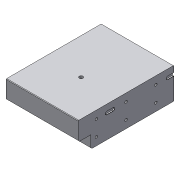
# Autodesk Inventor part: BC-10010
Saved by Autodesk Inventor 2016 (Build 200138000, 138)
## iProperties
Created: 2015-10-07
Part Number: BC-10010
Project: DIPOLO BC-3T- SIRIUS
Cost Center: 1504002005
Material: Alumínio 7075
Document SubType Name: Modeling
Designer: reinaldo.basilio
Mass: 37073.4 g
Surface Area: 4103.36 cm^2
Volume: 13193.4 cm^3
Density: 2.81 g/cm^3
Appearance: Aluminum - Flat
Description: Espaçador da metade superior e inferior do dipolo.
RuleStatus: InUse
AfterMaterialChange0: file://_iMaterial
AfterAnyiPropertyChange0: file://_iMaterial
AfterDocNew0: file://_Naming_par
AfterDocNew1: file://_NameStart
AfterDocNew2: file://_NameStart1
AfterDocNew3: file://_Materiais
DocNumber: XXXXX-XXX-XXXX-00-001.ipt
Folder: .
Title: DIPOLO BC-3T- SIRIUS
Author: reinaldo.basilio
Subject: BC-10010
Autodesk Inventor part; units mm, degrees
ref_plane "YZ Plane" through (0, 0, 0) normal (1, 0, 0) x (0, 1, 0)
ref_plane "XZ Plane" through (0, 0, 0) normal (0, 1, 0) x (-1, 0, 0)
ref_plane "XY Plane" through (0, 0, 0) normal (0, 0, 1) x (1, 0, 0)
sketch "Sketch5" plane through (0, 0, 0) normal (0, 1, 0) x (-1, 0, 0)
  line L0 (452.5, 48) -> (452.5, 173)
  line L1 (117.5, 98) -> (117.5, 48)
  line L2 (117.5, 48) -> (452.5, 48)
  line L3 (67.5, 173) -> (67.5, 98)
  line L4 (67.5, 98) -> (117.5, 98)
  line L5 (67.5, 173) -> (452.5, 173)
  dimension "d8" = 125
  dimension "d13" = 385
  dimension "d18" = 50
  dimension "d42" = 50
  constraints: 12 end point, 2 horizontal, 2 perpendicular, 2 vertical
  measures "d8" distance of L0.start L0.end
  measures "d13" distance of L3.start L0.end
  measures "d18" distance of L1.start L1.end
  measures "d42" distance of L3.end L1.start
extrude "Extrusion5" add sketch "Sketch5" along normal blind 291
sketch "Sketch6" plane through (0, 291, 0) normal (0, 1, 0) x (1, 0, 0)
  line L0 (-452.5, -173) -> (-67.5, -173) projected
  line L1 (-117.5, -48) -> (-452.5, -48) projected
  circle A0 centre (-140, -141.75) radius 6
  circle A1 centre (-140, -79.25) radius 6
  circle A2 centre (-260, -141.75) radius 6
  circle A3 centre (-260, -79.25) radius 6
  circle A4 centre (-380, -141.75) radius 6
  circle A5 centre (-380, -79.25) radius 6
  line L2 (-452.5, -48) -> (-452.5, -173) projected
  line L3 (-67.5, -173) -> (-67.5, -98) projected
  point P0 (0, 0)
  point P1 (-260, -173)
  dimension "d19" = 12
  dimension "d20" = 120
  dimension "d21" = 385
  dimension "d22" = 125
  dimension "d23" = 120
  dimension "d24" = 62.5
  dimension "d25" = 31.25
  dimension "d26" = 31.25
  dimension "d41" = 72.5
  dimension "d61" = 72.5
  dimension "d62" = 192.5
  constraints: 6 centre point, 5 equal radius, 4 horizontal alignment, 4 vertical alignment, 1 midpoint
  measures "d19" diameter of A0
  measures "d20" distance of A2.centre A0.centre
  measures "d21" distance of L0.start L0.end
  measures "d22" distance of L1.end L0.start
  measures "d23" distance of A4.centre A2.centre
  measures "d24" distance of A5.centre A4.centre
  measures "d25" distance from line of L0 A4.centre
  measures "d26" distance from line of L1 A5.centre
  measures "d41" distance from line of L2 A4.centre
  measures "d61" distance from line of L3 A0.centre
  measures "d62" distance from line of A3.centre L2
hole "Hole1" at (-140, 291, 141.75) at (-260, 291, 141.75) at (-380, 291, 141.75) at (-380, 291, 79.25) at (-260, 291, 79.25) at (-140, 291, 79.25) direction (0, -1, 0) diameter 10.106 depth 35 tip angle 118 thread size "M12x1.75" class "6H" standard "ISO Metric profile"
sketch "Sketch7" plane through (0, 0, 0) normal (0, -1, 0) x (1, 0, 0)
  circle A0 centre (-380, 141.75) radius 5.053
  circle A1 centre (-380, 79.25) radius 5.053
  circle A2 centre (-260, 141.75) radius 5.053
  circle A3 centre (-260, 79.25) radius 5.053
  circle A4 centre (-140, 141.75) radius 5.053
  circle A5 centre (-140, 79.25) radius 5.053
  circle A6 centre (-140, 141.75) radius 5.053 projected
  circle A7 centre (-140, 79.25) radius 5.053 projected
  circle A8 centre (-260, 79.25) radius 5.053 projected
  circle A9 centre (-260, 141.75) radius 5.053 projected
  circle A10 centre (-380, 141.75) radius 5.053 projected
  circle A11 centre (-380, 79.25) radius 5.053 projected
  point P0 (0, 0)
  constraints: 12 concentric, 6 centre point
hole "Hole2" at (-380, 0, 141.75) at (-380, 0, 79.25) at (-260, 0, 79.25) at (-260, 0, 141.75) at (-140, 0, 141.75) at (-140, 0, 79.25) direction (0, 1, 0) diameter 10.106 depth 35 tip angle 118 thread size "M12x1.75" class "6H" standard "ISO Metric profile"
chamfer "Chamfer1" distance 5 angle 45 2 edges at (-67.5, 145.5, 98) (-117.5, 145.5, 48)
sketch "Sketch8" plane through (0, 291, 0) normal (0, 1, 0) x (1, 0, 0)
  line L0 (-182.5, -141.75) -> (-207.5, -141.75) construction
  line L1 (-182.5, -135.75) -> (-207.5, -135.75)
  line L2 (-207.5, -147.75) -> (-182.5, -147.75)
  arc A0 (-182.5, -147.75) -> (-182.5, -135.75) centre (-182.5, -141.75) ccw
  arc A1 (-207.5, -135.75) -> (-207.5, -147.75) centre (-207.5, -141.75) ccw
  line L3 (-427.5, -141.75) -> (-452.5, -141.75) construction
  line L4 (-427.5, -135.75) -> (-452.5, -135.75)
  line L5 (-452.5, -147.75) -> (-427.5, -147.75)
  arc A2 (-427.5, -147.75) -> (-427.5, -135.75) centre (-427.5, -141.75) ccw
  arc A3 (-452.5, -135.75) -> (-452.5, -147.75) centre (-452.5, -141.75) ccw
  line L6 (-452.5, -48) -> (-452.5, -173) projected
  circle A4 centre (-260, -141.75) radius 5.053 projected
  point P0 (0, 0)
  point P1 (-440, -141.75)
  point P2 (-195, -141.75)
  point P3 (-440, -141.75)
  point P4 (-195, -147.75)
  point P5 (-195, -141.75)
  dimension "d46" = 12
  dimension "d47" = 12
  dimension "d48" = 25
  dimension "d49" = 25
  dimension "d58" = 12.5
  dimension "d60" = 257.5
  constraints: 16 end point, 8 point on circle, 8 tangent, 4 centre point, 4 midpoint, 2 parallel, 2 point on line, 1 coincident, 1 horizontal, 1 horizontal alignment, 1 vertical alignment
  measures "d46" distance between parallel lines of L1 L2
  measures "d47" distance between parallel lines of L4 L5
  measures "d48" distance of L0.start L0.end
  measures "d49" distance of L3.start L3.end
  measures "d58" distance from line of L6 point (-440, -141.75)
  measures "d60" distance from line of L6 point (-195, -141.75)
extrude "Extrusion6" cut sketch "Sketch8" against normal blind 5 contours A0 L2 A1 L1 | A2 L5 L6 L4 | L6 A3
sketch "Sketch9" plane through (0, 0, 0) normal (0, -1, 0) x (1, 0, 0)
  line L0 (-452.5, 141.75) -> (-427.5, 141.75) construction
  line L1 (-452.5, 135.75) -> (-427.5, 135.75)
  line L2 (-427.5, 147.75) -> (-452.5, 147.75)
  arc A0 (-452.5, 147.75) -> (-452.5, 135.75) centre (-452.5, 141.75) ccw
  arc A1 (-427.5, 135.75) -> (-427.5, 147.75) centre (-427.5, 141.75) ccw
  line L3 (-207.5, 141.75) -> (-182.5, 141.75) construction
  line L4 (-207.5, 135.75) -> (-182.5, 135.75)
  line L5 (-182.5, 147.75) -> (-207.5, 147.75)
  arc A2 (-207.5, 147.75) -> (-207.5, 135.75) centre (-207.5, 141.75) ccw
  arc A3 (-182.5, 135.75) -> (-182.5, 147.75) centre (-182.5, 141.75) ccw
  arc A4 (-427.5, 135.75) -> (-427.5, 147.75) centre (-427.5, 141.75) ccw projected
  arc A5 (-207.5, 147.75) -> (-207.5, 135.75) centre (-207.5, 141.75) ccw projected
  arc A6 (-182.5, 135.75) -> (-182.5, 147.75) centre (-182.5, 141.75) ccw projected
  line L6 (-452.5, 48) -> (-452.5, 173) projected
  point P0 (0, 0)
  point P1 (-440, 141.75)
  point P2 (-195, 141.75)
  dimension "d76" = 25
  dimension "d77" = 25
  dimension "d78" = 12.5
  constraints: 16 end point, 8 point on circle, 8 tangent, 4 centre point, 4 concentric, 2 midpoint, 2 parallel, 2 point on line, 1 horizontal
  measures "d76" distance of L3.start L3.end
  measures "d77" distance of L0.start L0.end
  measures "d78" distance from line of point (-440, 141.75) L6
extrude "Extrusion7" cut sketch "Sketch9" against normal blind 5
sketch "Sketch10" plane through (-452.5, 0, 48) normal (0, 0, -1) x (-1, 0, 0)
  line L0 (0, 0) -> (0, 291) projected
  line L1 (-330, 291) -> (0, 291) projected
  circle A0 centre (-295, 145.5) radius 5
  circle A1 centre (-165, 145.5) radius 5
  circle A2 centre (-35, 145.5) radius 5
  point P0 (-452.5, 0)
  point P1 (0, 145.5)
  point P2 (-165, 291)
  dimension "d63" = 130
  dimension "d64" = 130
  dimension "d65" = 10
  constraints: 3 centre point, 3 horizontal alignment, 2 equal radius, 2 midpoint, 1 vertical alignment
  measures "d63" distance of A1.centre A0.centre
  measures "d64" distance of A2.centre A1.centre
  measures "d65" diameter of A0
hole "Hole3" at (-157.5, 145.5, 48) at (-287.5, 145.5, 48) at (-417.5, 145.5, 48) direction (0, 0, 1) diameter 8.376 depth 25 tip angle 118 thread size "M10x1.5" class "6H" standard "ISO Metric profile"
chamfer "Chamfer2" distance 0.5 angle 45 14 edges at (-195, 291, 147.75) (-213.5, 291, 141.75) (-195, 291, 135.75) (-176.5, 291, 141.75) (-440, 291, 147.75) (-440, 291, 135.75) (-421.5, 291, 141.75) (-213.5, 0, 141.75) (-195, 0, 147.75) (-176.5, 0, 141.75) (-195, 0, 135.75) (-440, 0, 147.75) (-421.5, 0, 141.75) (-440, 0, 135.75)
chamfer "Chamfer3" distance 2 angle 45 3 edges at (-67.5, 145.5, 173) (-452.5, 145.5, 173) (-452.5, 145.5, 48)
sketch "Sketch11" plane through (-450.5, 0, 173) normal (0, 0, 1) x (1, 0, 0)
  circle A0 centre (226.5, 145.5) radius 7.5
  line L0 (-2, 291) -> (-2, 0) projected
  point P0 (450.5, 0)
  point P1 (-2, 145.5)
  dimension "d82" = 228.5
  dimension "d83" = 15
  constraints: 1 centre point, 1 horizontal alignment, 1 midpoint
  measures "d82" distance from line of A0.centre L0
  measures "d83" diameter of A0
hole "Hole4" at (-224, 145.5, 173) direction (0, 0, -1) diameter 15 end through all
sketch "Sketch12" plane through (-452.5, 286, 135.75) normal (-1, 0, 0) x (0, 0, 1)
  line L0 (-85.75, -286) -> (-85.75, 5) projected
  line L1 (-85.75, -286) -> (-0.5, -286) projected
  line L2 (-85.75, 5) -> (-0.5, 5) projected
  circle A0 centre (-65.25, -105.5) radius 5
  circle A1 centre (14.75, -105.5) radius 5
  circle A2 centre (-65.25, -175.5) radius 5
  circle A3 centre (14.75, -175.5) radius 5
  line L3 (-85.75, -140.5) -> (-93.0771, -140.5)
  line L4 (37.25, -286) -> (37.25, 5) projected
  line L5 (-87.75, 5) -> (-87.75, -286) projected
  point P0 (-135.75, -286)
  dimension "d91" = 10
  dimension "d92" = 80
  dimension "d94" = 70
  dimension "d96" = 35
  dimension "d97" = 125
  dimension "d99" = 22.5
  dimension "d100" = 110.5
  dimension "d101" = 110.5
  constraints: 4 centre point, 3 equal radius, 2 end point, 2 horizontal alignment, 2 vertical alignment, 1 horizontal, 1 midpoint
  measures "d91" diameter of A0
  measures "d92" distance of A1.centre A0.centre
  measures "d94" distance of A2.centre A0.centre
  measures "d96" vertical distance of L3.start A0.centre
  measures "d97" distance between parallel lines of L4 L5
  measures "d99" distance from line of L5 A0.centre
  measures "d100" distance from line of L2 A0.centre
  measures "d101" distance from line of L1 A2.centre
hole "Hole5" at (-452.5, 180.5, 150.5) at (-452.5, 180.5, 70.5) at (-452.5, 110.5, 150.5) at (-452.5, 110.5, 70.5) direction (1, 0, 0) diameter 8.376 depth 25 tip angle 118 thread size "M10x1.5" class "6H" standard "ISO Metric profile"
equation "\"d20\" = d23"
equation "\"d25\" = -0.5 * d24 + 0.5 * d22"
equation "\"d47\" = d46"
equation "\"d49\" = d48"
equation "\"d64\" = d63"
equation "\"d96\" = 0.5 * d94"
equation "\"d99\" = -0.5 * d92 + 0.5 * d97"
body "Solid5"
